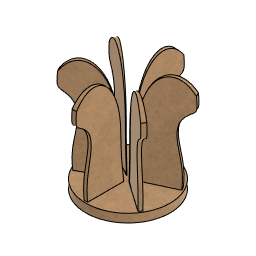
袜子晾晒架 v2 (Autodesk Fusion 360 design; units mm, degrees)
Autodesk Fusion 360 part; units mm, degrees
sketch "草图1" plane through (0, 0, 0) normal (0, 0, 1) x (1, 0, 0)
  circle A0 centre (0, 0) radius 100
  dimension "d1" = 200
  constraint coincident A0.centre origin
  measures "d1" diameter of A0
extrude "拉伸1" add sketch "草图1" along normal blind 20 makes body 1
sketch "草图3" plane through (0, 0, 0) normal (1, 0, 0) x (0, 1, 0)
  line L0 (100, 20) -> (-100, 20)
  line L1 (100, 20) -> (10, 20)
  spline S0 degree 5 poles (10, 20) (10.2597, 22.5752) (10.8069, 27.8082) (11.7109, 35.9052) (13.0305, 47.1717) (14.6043, 61.9126) (15.824, 77.1805) (16.5201, 92.8974) (16.7606, 109.0979) (16.966, 125.9843) (17.7481, 143.7421) (19.7767, 162.4167) (23.6163, 181.6692) (29.6192, 200.7933) (37.6824, 218.1009) (47.3552, 232.0036) (58.1511, 241.9284) (69.5322, 247.6886) (81.0119, 249.453) (92.2139, 247.4597) (102.9283, 241.8857) (111.0293, 234.6598) (116.828, 227.715) (120.5712, 222.41) (122.4122, 219.5887) knots 0 0 0 0 0 0 0.05 0.1 0.15 0.2 0.25 0.3 0.35 0.4 0.45 0.5 0.55 0.6 0.65 0.7 0.75 0.8 0.85 0.9 0.95 1 1 1 1 1 1
  line L2 (6.4538, -15.1595) -> (13.5462, 55.1595)
  line L3 (13.3756, 156.8128) -> (46.6244, 243.1872)
  spline S1 degree 5 poles (96.0083, 19.3299) (96.2262, 21.4899) (96.6233, 25.8261) (97.1033, 32.379) (97.4796, 41.2499) (97.3531, 52.7597) (96.4813, 64.9181) (94.8075, 77.9078) (92.4588, 91.785) (89.8228, 106.4094) (87.6767, 121.3381) (86.9933, 135.9116) (88.6109, 149.392) (93.021, 161.0856) (99.9354, 170.466) (108.3149, 177.3171) (115.2139, 181.8306) (119.6773, 185.0188) (122.0659, 188.2207) (123.1731, 192.6832) (123.4837, 199.1188) (123.289, 206.111) (122.9323, 212.4326) (122.6011, 217.1238) (122.4122, 219.5887) knots 0 0 0 0 0 0 0.05 0.1 0.15 0.2 0.25 0.3 0.35 0.4 0.45 0.5 0.55 0.6 0.65 0.7 0.75 0.8 0.85 0.9 0.95 1 1 1 1 1 1
  line L4 (92.4621, -15.8295) -> (99.5545, 54.4894)
  line L5 (78.0607, 151.553) -> (132.3507, 197.4952)
  point P0 (16.375, 91.9339)
  point P1 (30, 200)
  point P2 (78.5459, 248.449)
  point P3 (121.7333, 188.5103)
  point P4 (105.2057, 174.5241)
  point P5 (91.8091, 95.3422)
  dimension "d4" = 90
  constraint coincident L0 L1.start
  constraint midpoint L1.end L2
  constraint midpoint P1 L3
  constraint midpoint S1.start L4
  constraint midpoint P4 L5
  constraint coincident P3 L5
  measures "d4" distance of L0.start L1.end
revolve "旋转1" add sketch "草图3" angle 5 about axis through (0, 0, 1.75) along (0, 0, -1) separate body makes body 2
pattern_circular "C-阵列1" count 6 over 360 about axis through (0, 0, 1.75) along (0, 0, 1) of bodies 2 makes body 3 at (-35.1371, 20.2864, 91.2944) makes body 4 at (-35.1371, -20.2864, 91.2944) makes body 5 at (0, -40.5729, 91.2944) makes body 6 at (35.1371, -20.2864, 91.2944) makes body 7 at (36.7715, 17.1468, 91.2944)
combine "合并1" operation add target body 1 tool bodies 2 3 4 5 6 7
